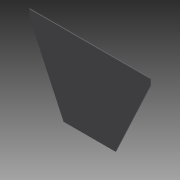
# Autodesk Inventor part: electrical board back
Saved by Autodesk Inventor 2012 (Build 160160000, 160)
## iProperties
Created: 2011-10-06
Part Number: electrical board back
Material: ABS Plastic
Document SubType Name: Modeling
Designer: Antonella
Mass: 534.136 g
Surface Area: 3227.61 cm^2
Volume: 503.902 cm^3
Density: 1.06 g/cm^3
Author: Antonella
Autodesk Inventor part; units mm, degrees
ref_plane "YZ Plane" through (0, 0, 0) normal (1, 0, 0) x (0, 1, 0)
ref_plane "XZ Plane" through (0, 0, 0) normal (0, 1, 0) x (-1, 0, 0)
ref_plane "XY Plane" through (0, 0, 0) normal (0, 0, 1) x (1, 0, 0)
sketch "Sketch1" plane through (0, 0, 0) normal (0, 0, 1) x (1, 0, 0)
  line L0 (-320.04, 0) -> (320.04, 0) projected
  line L1 (0, -340.36) -> (0, 86.36) projected
  line L2 (-228.6, 25.4) -> (228.6, 25.4)
  line L3 (-98.425, -279.4) -> (98.425, -279.4)
  line L4 (-228.6, 0) -> (-98.425, -279.4)
  line L5 (228.6, 0) -> (98.425, -279.4)
  line L6 (228.6, 0) -> (228.6, 25.4)
  line L7 (-228.6, 0) -> (-228.6, 25.4)
  point P0 (0, 0)
  point P1 (0, 25.4)
  point P2 (0, -279.4)
  point P3 (0, 25.4)
  dimension "d0" = 196.85
  dimension "d2" = 304.8
  dimension "d7" = 25.4
  dimension "d8" = 457.2
  constraints: 12 end point, 3 midpoint, 3 parallel, 3 vertical alignment, 2 perpendicular, 1 point on line
  measures "d0" distance of L3.start L3.end
  measures "d2" distance between parallel lines of L2 L3
  measures "d7" distance of L4.start L2.start
  measures "d8" distance of L2.start L2.end
extrude "Extrusion1" add sketch "Sketch1" along normal mid plane 3.175
body "Solid1"
